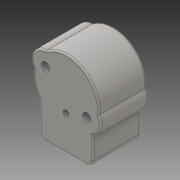
# Autodesk Inventor part: 15-697867-75
Saved by Autodesk Inventor 2016 SP1 (Build 200210100, 210)
## iProperties
Category: Control System
Company: Autodesk Inc.
Created: 2015-12-10
Part Number: 15-697867-75
Material: Generic
Document SubType Name: Modeling
Designer: Autodesk Inc.
Density: 1 g/cm^3
Appearance: Default
Catalog Web Link: http://www.ctr-electronics.com/srx-magnetic-encoder.html#product_tabs_technical_resources
Vendor: CTR Electronics
Author: Autodesk Inc.
Autodesk Inventor part; units mm, degrees
ref_plane "YZ Plane" through (0, 0, 0) normal (1, 0, 0) x (0, 1, 0)
ref_plane "XZ Plane" through (0, 0, 0) normal (0, 1, 0) x (-1, 0, 0)
ref_plane "XY Plane" through (0, 0, 0) normal (0, 0, 1) x (1, 0, 0)
sketch "Sketch1" plane through (0, 0, 0) normal (0, 1, 0) x (-1, 0, 0)
  line L0 (0, 0) -> (0, -21.748)
  line L1 (26.908, 0) -> (26.908, -21.748)
  line L2 (0, 0) -> (26.908, 0)
  line L3 (26.908, -21.748) -> (0, -21.748)
  circle A0 centre (16.637, -10.874) radius 7.442 construction
  line L4 (26.908, 0.5867) -> (26.908, -22.1122) construction
  line L5 (26.908, -22.1122) -> (-0.2229, -22.1122) construction
  line L6 (-0.2229, -22.1122) -> (-0.2229, 0.5867) construction
  line L7 (-0.2229, 0.5867) -> (26.908, 0.5867) construction
  arc A1 (24.7169, -4.533) -> (17.9518, -0.6875) centre (20.3146, -4.4042) ccw
  arc A2 (8.9733, -19.2168) -> (15.3222, -21.0605) centre (12.9594, -17.3438) ccw
  arc A3 (17.9518, -0.6875) -> (10.6061, -2.56) centre (16.637, -10.874) ccw
  arc A4 (15.3222, -21.0605) -> (24.7169, -4.533) centre (16.637, -10.874) ccw
  line L8 (10.6061, -2.56) -> (0, -2.56)
  line L9 (0, -2.56) -> (0, -19.2168)
  line L10 (0, -2.56) -> (0, -19.2168)
  line L11 (0, -19.2168) -> (8.9733, -19.2168)
  circle A5 centre (20.3146, -4.4042) radius 1.321
  circle A6 centre (12.9594, -17.3438) radius 1.321
  circle A7 centre (10.8743, -10.874) radius 0.889
  point P0 (0, -10.874)
  dimension "d0" = 26.908
  dimension "d1" = 21.748
  dimension "d2" = 16.637
  dimension "d3" = 7.442
  dimension "d21" = 2.642
  dimension "d22" = 1.778
  constraints: 16 end point, 10 point on circle, 8 centre point, 4 coincident, 3 equal radius, 3 horizontal, 3 tangent, 2 parallel, 2 point on line, 2 vertical, 1 collinear, 1 horizontal alignment, 1 midpoint, 1 perpendicular, 2 other
  measures "d0" distance between parallel lines of L1 L0
  measures "d1" distance of L1.start L1.end
  measures "d2" distance from line of point (16.637, -10.874) L0
  measures "d3" radius of A0
  measures "d21" diameter of A5
  measures "d22" diameter of A7
extrude "Extrusion1" add sketch "Sketch1" along normal blind 15 contours L8 A3 A1 A4 A2 L11 L0
fillet "Fillet1" radius 2 2 edges at (0, 7.5, -2.56) (0, 7.5, -19.2168)
fillet "Fillet2" radius 0.5 18 edges at (-14.0999, 0, -0.9213) (-0.5858, 0, -3.1458) (0, 0, -10.8884) (-0.5858, 0, -18.631) (-5.4867, 0, -19.2168) (-6.3031, 0, -2.56) (-11.7312, 0, -21.5733) (-25.5663, 0, -15.9496) (-22.491, 0, -0.5753) (-6.3031, 15, -2.56) (0, 15, -10.8884) (-0.5858, 15, -18.631) (-5.4867, 15, -19.2168) (-0.5858, 15, -3.1458) (-14.0999, 15, -0.9213) (-22.491, 15, -0.5753) (-25.5663, 15, -15.9496) (-11.7312, 15, -21.5733)
body "Solid1"
